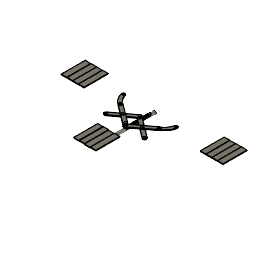
KOM_tonfa_shield_toy (Autodesk Fusion 360 design; units mm, degrees)
Autodesk Fusion 360 part; units mm, degrees
sketch "Sketch1" plane through (0, 0, 0) normal (0, 0, 1) x (1, 0, 0)
  circle A0 centre (0, 0) radius 10
  circle A1 centre (0, 0) radius 20
  dimension "d1" = 20
  dimension "d2" = 40
  constraint coincident A0.centre A1.centre
  constraint concentric A0 A1
  measures "d1" diameter of A0
  measures "d2" diameter of A1
extrude "Extrude1" add sketch "Sketch1" along normal blind 500 makes body 1
sketch "Sketch2" plane through (0, 0, 0) normal (0, 1, 0) x (1, 0, 0)
  line L0 (0, 0) -> (0, -65) construction
  line L1 (-15, -65) -> (-15, -365)
  arc A0 (-15, -365) -> (15, -365) centre (0, -365) ccw
  line L2 (15, -365) -> (15, -65)
  arc A1 (15, -65) -> (-15, -65) centre (0, -65) ccw
  line L3 (0, -65) -> (0, -365) construction
  dimension "d5" = 65
  dimension "d6" = 300
  dimension "d7" = 30
  constraint vertical L0
  constraint tangent L1 A0
  constraint tangent A0 L2
  constraint parallel L1 L2
  constraint tangent L2 A1
  constraint tangent L1 A1
  constraint parallel L0 L3
  constraint coincident L0.end A1.centre
  measures "d5" distance of L0.start L0.end
  measures "d6" distance of L0.end A0.centre
  measures "d7" diameter of A0
extrude "Extrude2" cut sketch "Sketch2" along normal blind 20 bodies 1
copy_body "Body->Comp1" bodies 1 removing the originals makes body 2 in component "Component"
sketch "Sketch3" plane through (0, 0, 0) normal (0, 1, 0) x (1, 0, 0)
  circle A0 centre (-75, 0) radius 15
  dimension "d10" = 30
  measures "d10" diameter of A0
sketch "Sketch4" plane through (0, 0, 0) normal (0, 1, 0) x (1, 0, 0)
  line L0 (100, -15) -> (400, -15)
  arc A0 (400, -15) -> (400, 15) centre (400, 0) ccw
  line L1 (400, 15) -> (100, 15)
  arc A1 (100, 15) -> (100, -15) centre (100, 0) ccw
  line L2 (100, 0) -> (400, 0) construction
  line L3 (100, -22.5) -> (400, -22.5)
  line L4 (400, 22.5) -> (100, 22.5)
  arc A2 (100, 22.5) -> (100, -22.5) centre (100, 0) ccw
  line L5 (100, 0) -> (400, 0) construction
  circle A3 centre (100, 0) radius 15
  circle A4 centre (250, 0) radius 15
  arc A5 (400, -22.5) -> (400, 22.5) centre (400, 0) ccw
  circle A6 centre (400, 0) radius 15
  dimension "d20" = 30
  dimension "d22" = 30
  dimension "d23" = 30
  dimension "d48" = 300
  dimension "d101" = 300
  dimension "d102" = 300
  dimension "d103" = 30
  constraint tangent L0 A0
  constraint tangent A0 L1
  constraint parallel L0 L1
  constraint tangent L1 A1
  constraint tangent L0 A1
  constraint horizontal L2
  constraint parallel L3 L4
  constraint tangent L4 A2
  constraint tangent L3 A2
  constraint coincident A0.centre L2.end
  constraint parallel L2 L5
  constraint coincident A1.centre L2.start
  constraint concentric A1 A3
  constraint concentric A0 A6
  measures "d20" diameter of A0
  measures "d22" diameter of A3
  measures "d23" diameter of A4
  measures "d48" distance of A1.centre A0.centre
  measures "d101" distance of L4.start L4.end
  measures "d102" distance of L3.start L3.end
  measures "d103" diameter of A6
extrude "Extrude4" add sketch "Sketch4" along normal blind 10 separate body contours L0 L1 A3 A4 | L0 L1 A4 A6 | L3 L4 A2 A5 makes body 3
copy_body "CopyPasteBodies1" bodies 3 makes body 4
move_body "Move1" bodies 4 to x (1, 0, 0) y (0, 1, 0) z (0, 0, 1) at (0, 0, 90)
copy_body "Body->Comp3" bodies 3 removing the originals makes body 5 in component "Component'"
copy_body "Body->Comp4" bodies 4 removing the originals makes body 6 in component "Component''"
copy_body "CopyPasteBodies3" bodies 5 body 5 seen with x (0.975479, 0, 0.220093) y (0, 1, 0) z (-0.220093, 0, 0.975479) at (-97.5479, 20, 42.9907) makes body 7
move_body "Move3" bodies 7 to x (1, 0, 0) y (0, 1, 0) z (0, 0, 1) at (0, 0, 300)
copy_body "CopyPasteBodies4" bodies 6 body 6 seen with x (-0.954914, 0, 0.296882) y (0, 1, 0) z (-0.296882, 0, -0.954914) at (122.2108, 30, 121.2541) makes body 8
move_body "Move4" bodies 8 to x (1, 0, 0) y (0, 1, 0) z (0, 0, 1) at (0, 0, 300)
copy_body "Body->Comp6" bodies 7 removing the originals makes body 9 in component "Component'''"
copy_body "Body->Comp7" bodies 8 removing the originals makes body 10 in component "Component''''"
extrude "Extrude5" add sketch "Sketch3" along normal blind 20 separate body makes body 11
copy_body "CopyPasteBodies7" bodies 11 makes body 12
move_body "Move7" bodies 12 to x (1, 0, 0) y (0, 1, 0) z (0, 0, 1) at (0, 0, 50)
copy_body "Body->Comp10" bodies 11 removing the originals makes body 13 in component "Component'''''"
copy_body "Body->Comp11" bodies 12 removing the originals makes body 14 in component "Component''''''"
extrude "Extrude6" add sketch "Sketch3" along normal blind 70 separate body makes body 15
copy_body "Body->Comp12" bodies 15 removing the originals makes body 16 in component "Component'''''''"
extrude "Extrude7" add sketch "Sketch3" along normal blind 60 separate body makes body 17
copy_body "Body->Comp13" bodies 17 removing the originals makes body 18 in component "Component''''''''"
sketch "Sketch5" plane through (0, 0, 0) normal (0, 1, 0) x (1, 0, 0)
  arc A0 (185, 150) -> (132.0288, 279.5893) centre (0, 150) ccw
  arc A1 (185, 150) -> (215, 150) centre (200, 150) ccw
  arc A2 (215, 150) -> (153.4389, 300.6038) centre (0, 150) ccw
  arc A3 (153.4389, 300.6038) -> (132.0288, 279.5893) centre (142.7339, 290.0965) ccw
  arc A4 (200, 150) -> (142.7339, 290.0965) centre (0, 150) ccw construction
  arc A5 (180, 150) -> (128.4605, 276.0869) centre (0, 150) ccw
  arc A6 (180, 150) -> (220, 150) centre (200, 150) ccw
  arc A7 (220, 150) -> (157.0073, 304.1062) centre (0, 150) ccw
  arc A8 (157.0073, 304.1062) -> (128.4605, 276.0869) centre (142.7339, 290.0965) ccw
  arc A9 (200, 150) -> (142.7339, 290.0965) centre (0, 150) ccw construction
  circle A10 centre (142.7339, 290.0965) radius 15
  circle A11 centre (200, 150) radius 15
  dimension "d120" = 30
  dimension "d121" = 30
  dimension "d132" = 200
  constraint tangent A0 A1
  constraint tangent A1 A2
  constraint tangent A2 A3
  constraint tangent A0 A3
  constraint tangent A5 A6
  constraint tangent A6 A7
  constraint tangent A7 A8
  constraint tangent A5 A8
  constraint coincident A0.centre A2.centre
  constraint coincident A3.centre A4.end
  constraint coincident A1.centre A4.start
  constraint concentric A8 A10
  constraint concentric A6 A11
  measures "d120" diameter of A10
  measures "d121" diameter of A11
  measures "d132" radius of A4
extrude "Extrude8" add sketch "Sketch5" along normal blind 10 separate body contours A0 A2 A10 A11 | A5 A6 A7 A8 makes body 19
copy_body "CopyPasteBodies8" bodies 19 makes body 20
move_body "Move8" bodies 20 to x (1, 0, 0) y (0, 1, 0) z (0, 0, 1) at (-80, 0, 0)
copy_body "Body->Comp14" bodies 19 removing the originals makes body 21 in component "Component'''''''''"
copy_body "Body->Comp15" bodies 20 removing the originals makes body 22 in component "Component''''''''''"
sketch "Sketch6" plane through (0, 0, 0) normal (0, 1, 0) x (1, 0, 0)
  line L0 (-250, -300) -> (-180, -300)
  line L1 (-180, -300) -> (-180, 0)
  line L2 (-180, 0) -> (-250, 0)
  line L3 (-250, 0) -> (-250, -300)
  dimension "d143" = 70
  dimension "d144" = 300
  constraint horizontal L0
  constraint vertical L1
  constraint horizontal L2
  constraint vertical L3
  measures "d143" distance of L0.start L0.end
  measures "d144" distance of L0.start L2.end
extrude "Extrude9" add sketch "Sketch6" along normal blind 7 separate body makes body 23
copy_body "Body->Comp16" bodies 23 removing the originals makes body 24 in component "Component'''''''''''"
component "Component'" placed x (-0.113624, 0, -0.993524) y (0, 1, 0) z (0.993524, 0, -0.113624) at (11.3624, 50, 464.3524)
component "Component''" placed x (-0.113624, 0, 0.993524) y (0, 1, 0) z (-0.993524, 0, -0.113624) at (134.8669, 30, -22.1833)
component "Component" placed x (1, 0, 0) y (0, 1, 0) z (0, 0, 1) at (0, 0, 0)
component "Component'''" placed x (0.329506, 0, 0.944154) y (0, 1, 0) z (-0.944154, 0, 0.329506) at (344.616, 0, -53.3268)
component "Component''''" placed x (-0.403461, 0, 0.914997) y (0, 1, 0) z (-0.914997, 0, -0.403461) at (299.8866, 10, 512.2632)
component "Component'''''" placed x (0.970124, 0, 0.24261) y (0, 1, 0) z (-0.24261, 0, 0.970124) at (55.7156, 40, 234.1672)
component "Component''''''" placed x (-0.959098, 0, -0.283075) y (0, 1, 0) z (0.283075, 0, -0.959098) at (-69.0424, 20, 242.6957)
component "Component'''''''" placed x (0, 0, -1) y (0, 1, 0) z (1, 0, 0) at (0, 0, 290)
component "Component''''''''" placed x (1, 0, 0) y (0, -1, 0) z (0, 0, -1) at (75, 60, 66.9429)
component "Component'''''''''" placed x (-0.83412, 0, -0.551583) y (0, 1, 0) z (0.551583, 0, -0.83412) at (244.9823, 50, -96.3027)
component "Component''''''''''" placed x (0.97984, 0, 0.199783) y (0, 1, 0) z (-0.199783, 0, 0.97984) at (-113.461, 30, 189.9449)
component "Component'''''''''''" placed x (1, 0, 0) y (0, 1, 0) z (0, 0, 1) at (0, 0, 0)
component "Component'''''''''''" placed x (1, 0, 0) y (0, 1, 0) z (0, 0, 1) at (-100, 0, 0)
component "Component'''''''''''" placed x (1, 0, 0) y (0, 1, 0) z (0, 0, 1) at (-200, 0, 0)
component "Component'''''''''''" placed x (1, 0, 0) y (0, 1, 0) z (0, 0, 1) at (-300, 0, 0)
component "Component'''''''''''" placed x (1, 0, 0) y (0, 1, 0) z (0, 0, 1) at (-400, 0, 0)
component "Component'''''''''''" placed x (1, 0, 0) y (0, 1, 0) z (0, 0, 1) at (-500, 0, 0)
component "Component'''''''''''" placed x (1, 0, 0) y (0, 1, 0) z (0, 0, 1) at (0, 0, 300)
component "Component'''''''''''" placed x (1, 0, 0) y (0, 1, 0) z (0, 0, 1) at (-100, 0, 300)
component "Component'''''''''''" placed x (1, 0, 0) y (0, 1, 0) z (0, 0, 1) at (-200, 0, 300)
component "Component'''''''''''" placed x (1, 0, 0) y (0, 1, 0) z (0, 0, 1) at (-300, 0, 300)
component "Component'''''''''''" placed x (1, 0, 0) y (0, 1, 0) z (0, 0, 1) at (-400, 0, 300)
component "Component'''''''''''" placed x (1, 0, 0) y (0, 1, 0) z (0, 0, 1) at (-500, 0, 300)
equation "d7 = d10"
equation "d20 = d7"
equation "d22 = d7"
equation "d23 = d7"
equation "d103 = d10"
equation "d120 = d10"
equation "d121 = d10"
